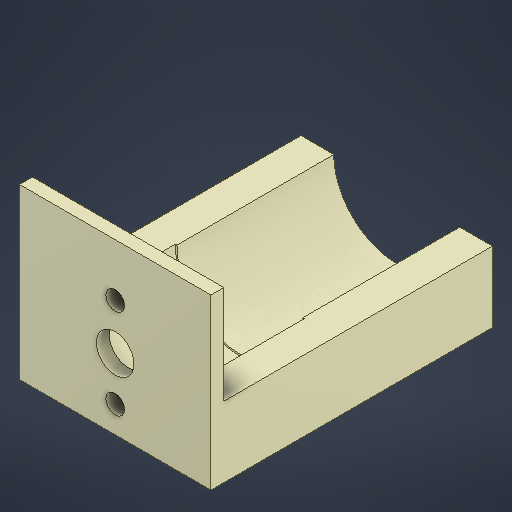
# Autodesk Inventor part: motor_holder
Saved by Autodesk Inventor 2026 (Build 300175050, 175E)
## iProperties
Created: 2025-06-04
Part Number: motor_holder
Material: Generic
Document SubType Name: Modeling
Designer: satom
Density: 1 g/cm^3
Appearance: Smooth - Ash
Author: satom
Autodesk Inventor part; units mm, degrees
ref_plane "YZ Plane" through (0, 0, 0) normal (1, 0, 0) x (0, 1, 0)
ref_plane "XZ Plane" through (0, 0, 0) normal (0, 1, 0) x (-1, 0, 0)
ref_plane "XY Plane" through (0, 0, 0) normal (0, 0, 1) x (1, 0, 0)
sketch "Sketch1" plane through (0, 0, 0) normal (0, 0, 1) x (1, 0, 0)
  line L0 (0, 0) -> (37.0648, 0)
  line L1 (37.0648, 0) -> (37.0648, 13.65)
  line L2 (0, 0) -> (0, 13.65)
  line L3 (0, 13.65) -> (6.35, 13.65)
  line L4 (37.0648, 13.65) -> (30.7148, 13.65)
  line L5 (18.5324, 0) -> (18.5324, 24.6661)
  line L6 (6.35, 13.65) -> (30.7148, 13.65) construction
  arc A0 (6.35, 13.65) -> (30.7148, 13.65) centre (18.5324, 13.65) ccw
  dimension "d0" = 37.0648
  dimension "d1" = 13.65
  dimension "d2" = 13.65
  dimension "d3" = 6.35
  dimension "d4" = 6.35
  dimension "d5" = 12.1824
  dimension "d6" = 13.65
  constraints: 14 end point, 3 horizontal, 2 midpoint, 2 point on circle, 2 vertical, 1 centre point, 1 perpendicular, 1 point on line
  measures "d0" distance of L0.start L0.end
  measures "d1" distance of L0.start L2.end
  measures "d2" distance of L0.end L1.end
  measures "d3" distance of L2.end L3.end
  measures "d4" distance of L1.end L4.end
  measures "d5" radius of A0
  measures "d6" distance from line of L0 A0.centre
extrude "Extrusion1" add sketch "Sketch1" along normal blind 30.365
sketch "Sketch2" plane through (0, 0, 30.365) normal (0, 0, 1) x (1, 0, 0)
  line L0 (0, 13.65) -> (0, 0) projected
  line L1 (0, 0) -> (37.0648, 0) projected
  line L2 (0, 0) -> (37.0648, 0)
  line L3 (37.0648, 0) -> (37.0648, 13.65)
  line L4 (0, 0) -> (0, 13.65)
  line L5 (0, 13.65) -> (6.042, 13.65)
  arc A0 (6.35, 13.65) -> (30.7148, 13.65) centre (18.5324, 13.65) ccw projected
  line L6 (6.35, 13.65) -> (30.7148, 13.65) construction
  line L7 (18.5324, 0) -> (18.5324, 13.65)
  line L8 (37.0648, 13.65) -> (31.0228, 13.65)
  arc A1 (6.042, 13.65) -> (31.0228, 13.65) centre (18.5324, 13.65) ccw
  dimension "d9" = 13.65
  dimension "d10" = 13.65
  dimension "d11" = 6.042
  dimension "d13" = 37.0648
  dimension "d15" = 6.042
  dimension "d16" = 12.4904
  constraints: 14 end point, 2 point on circle, 2 symmetric about line, 1 centre point, 1 coincident, 1 collinear, 1 horizontal, 1 midpoint, 1 vertical
  measures "d9" distance of L0.start L0.end
  measures "d10" distance of L1.end L3.end
  measures "d11" distance of L4.end L5.end
  measures "d13" distance of L0.end L1.end
  measures "d15" distance of L8.start L8.end
  measures "d16" radius of A1
extrude "Extrusion2" add sketch "Sketch2" along normal blind 21.635
sketch "Sketch3" plane through (0, 0, 52) normal (0, 0, 1) x (1, 0, 0)
  line L0 (0, 0) -> (37.0648, 0)
  line L1 (0, 0) -> (37.0648, 0)
  line L2 (37.0648, 0) -> (37.0648, 32.7)
  line L3 (37.0648, 32.7) -> (0, 32.7)
  line L4 (0, 32.7) -> (0, 0)
  line L5 (18.5324, 32.7) -> (18.5324, 0)
  line L6 (0, 0) -> (37.0648, 0) projected
  circle A0 centre (18.5324, 22.54) radius 1.8
  circle A1 centre (18.5324, 13.65) radius 3.625
  circle A2 centre (18.5324, 5.141) radius 1.8
  dimension "d19" = 37.0648
  dimension "d20" = 32.7
  dimension "d21" = 7.25
  dimension "d22" = 3.6
  dimension "d23" = 3.6
  dimension "d24" = 13.65
  dimension "d25" = 8.509
  dimension "d26" = 8.89
  constraints: 12 end point, 3 centre point, 3 point on line, 2 horizontal, 2 midpoint, 2 parallel, 1 perpendicular
  measures "d19" distance of L0.start L0.end
  measures "d20" distance of L1.end L2.end
  measures "d21" diameter of A1
  measures "d22" diameter of A2
  measures "d23" diameter of A0
  measures "d24" distance from line of L0 A1.centre
  measures "d25" distance of A1.centre A2.centre
  measures "d26" distance of A0.centre A1.centre
extrude "Extrusion3" add sketch "Sketch3" along normal blind 2.5 contours L4 L3 L5 A0 A1 A2 L0 | L5 A2 A1 A0 L3 L2 L0
sketch "Sketch4" plane through (0, 0, 0) normal (0, -1, 0) x (1, 0, 0)
  circle A0 centre (31.9848, 48.15) radius 2
  circle A1 centre (5.08, 48.15) radius 2
  circle A2 centre (31.9848, 6.35) radius 2
  circle A3 centre (5.08, 6.35) radius 2
  line L0 (0, 54.5) -> (37.0648, 54.5) projected
  line L1 (37.0648, 0) -> (37.0648, 54.5) projected
  line L2 (0, 0) -> (37.0648, 0) projected
  line L3 (0, 0) -> (0, 54.5) projected
  dimension "d29" = 4
  dimension "d30" = 4
  dimension "d32" = 4
  dimension "d33" = 4
  dimension "d34" = 6.35
  dimension "d35" = 5.08
  dimension "d36" = 5.08
  dimension "d37" = 6.35
  dimension "d38" = 6.35
  dimension "d39" = 5.08
  dimension "d40" = 6.35
  dimension "d41" = 5.08
  dimension "d42" = 26.9048
  dimension "d43" = 41.8
  constraints: 4 centre point
  measures "d29" diameter of A0
  measures "d30" diameter of A2
  measures "d32" diameter of A3
  measures "d33" diameter of A1
  measures "d34" distance from line of A0.centre L0
  measures "d35" distance from line of L1 A0.centre
  measures "d36" distance from line of L1 A2.centre
  measures "d37" distance from line of L2 A2.centre
  measures "d38" distance from line of L2 A3.centre
  measures "d39" distance from line of L3 A3.centre
  measures "d40" distance from line of L0 A1.centre
  measures "d41" distance from line of L3 A1.centre
  measures "d42" distance between centres of A0 A1
  measures "d43" distance of A3.centre A1.centre
extrude "Extrusion4" cut sketch "Sketch4" against normal blind 7 contours A0 | A1 | A2 | A3
equation "\"d2\" = d1"
body "Solid1"
